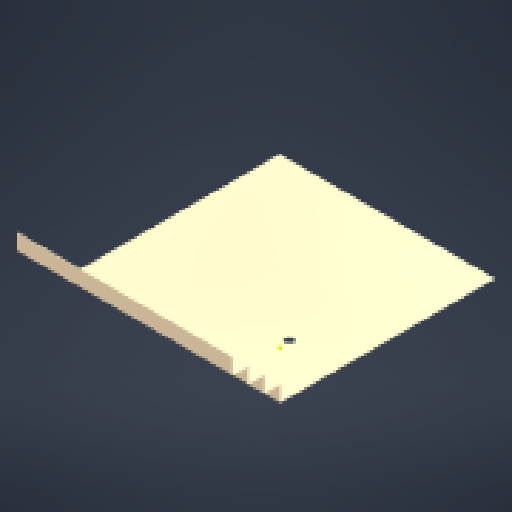
# Autodesk Inventor part: Floor, Shower
Saved by Autodesk Inventor 2026 (Build 300175000, 175)
## iProperties
Created: 2025-11-08
Part Number: Floor, Shower
Material: Polyethylene, High Density
Document SubType Name: Sheet Metal
Designer: Brandon Portillo
Density: 0.952 g/cm^3
Sheet Metal Rule: Default
Appearance: Smooth - Off-White
Author: Brandon Portillo
Autodesk Inventor part; units mm, degrees
ref_plane "YZ Plane" through (0, 0, 0) normal (1, 0, 0) x (0, 1, 0)
ref_plane "XZ Plane" through (0, 0, 0) normal (0, 1, 0) x (-1, 0, 0)
ref_plane "XY Plane" through (0, 0, 0) normal (0, 0, 1) x (1, 0, 0)
sketch "Sketch1" plane through (0, 0, 0) normal (0, 1, 0) x (-1, 0, 0)
  line L0 (0, 0) -> (1000, 0)
  line L1 (1000, 0) -> (1000, -1000)
  line L2 (1000, -1000) -> (0, -1000)
  line L3 (0, -1000) -> (0, 0)
  dimension "d0" = 1000
  dimension "d1" = 1000
  measures "d0" distance of L1.end L2.end
  measures "d1" distance of L0.end L1.end
extrude "Plate1" add sketch "Sketch1" along normal blind 3.048
sketch "Sketch2" plane through (0, 3.048, 0) normal (0, 1, 0) x (1, 0, 0)
  line L0 (-1000, 0) -> (0, 0) projected
  line L1 (0, 0) -> (-226.9109, 0)
  line L2 (-226.9109, 0) -> (-226.9109, 273.104)
  line L3 (-226.9109, 273.104) -> (0, 273.104)
  line L4 (0, 273.104) -> (0, 0)
  circle A0 centre (-226.9109, 273.104) radius 19.05
  dimension "d3" = 38.1
  constraints: 8 end point, 2 coincident, 2 parallel, 1 centre point, 1 horizontal, 1 perpendicular
  measures "d3" diameter of A0
extrude "Cut1" cut sketch "Sketch2" against normal blind 3.048 contours A0 L3 L2 | L2 L3 A0
sketch "Sketch3" plane through (0, 0, -3.048) normal (0, 0, 1) x (1, 0, 0)
  line L0 (-1000, 0) -> (0, 0)
  line L1 (0, 0) -> (0, 76.2)
  line L2 (0, 76.2) -> (-1000, 76.2)
  line L3 (-1000, 76.2) -> (-1000, 0)
  constraints: 6 end point, 1 horizontal, 1 perpendicular, 1 vertical
edge flange "Flange1" height 76.2 angle 90 thickness 3.048 bend radius 3.048 thickness toward (0, 0, 1) relief tear relief width 3.048 relief depth 1.524 edges at (-500, 3.048, 0) wall of the first edge with corners at (-1000, 0, -3.048) (0, 0, -3.048) (0, 76.2, -3.048) (-1000, 76.2, -3.048)
bend "Bend1"
corner "Corner1"
sketch "Sketch4" plane through (-1000, 73.152, -3.048) normal (0, 1, 0) x (-1, 0, 0)
  line L0 (-1000, 0) -> (0, 0)
  line L1 (0, 0) -> (0, 76.2)
  line L2 (0, 76.2) -> (-1000, 76.2)
  line L3 (-1000, 76.2) -> (-1000, 0)
  constraints: 6 end point, 1 horizontal, 1 perpendicular, 1 vertical
edge flange "Flange2" height 76.2 angle 90 thickness 3.048 bend radius 3.048 thickness toward (0, 1, 0) relief tear relief width 3.048 relief depth 1.524 edges at (-500, 76.2, 0) wall of the first edge with corners at (0, 73.152, -3.048) (-1000, 73.152, -3.048) (-1000, 73.152, 73.152) (0, 73.152, 73.152)
bend "Bend2"
corner "Corner2"
sketch "Sketch5" plane through (0, 73.152, 70.104) normal (0, 0, 1) x (1, 0, 0)
  line L0 (-1000, 0) -> (0, 0)
  line L1 (0, 0) -> (0, 76.2)
  line L2 (0, 76.2) -> (-1000, 76.2)
  line L3 (-1000, 76.2) -> (-1000, 0)
  constraints: 6 end point, 1 horizontal, 1 perpendicular, 1 vertical
edge flange "Flange3" height 76.2 angle 90 thickness 3.048 bend radius 3.048 thickness toward (0, 0, 1) relief tear relief width 3.048 relief depth 1.524 edges at (-500, 76.2, 73.152) wall of the first edge with corners at (-1000, 73.152, 70.104) (0, 73.152, 70.104) (0, 149.352, 70.104) (-1000, 149.352, 70.104)
bend "Bend3"
corner "Corner3"
sketch "Sketch6" plane through (-1000, 146.304, 70.104) normal (0, 1, 0) x (-1, 0, 0)
  line L0 (-1000, 0) -> (0, 0)
  line L1 (0, 0) -> (0, 76.2)
  line L2 (0, 76.2) -> (-1000, 76.2)
  line L3 (-1000, 76.2) -> (-1000, 0)
  constraints: 6 end point, 1 horizontal, 1 perpendicular, 1 vertical
edge flange "Flange4" height 76.2 angle 90 thickness 3.048 bend radius 3.048 thickness toward (0, 1, 0) relief tear relief width 3.048 relief depth 1.524 edges at (-500, 149.352, 73.152) wall of the first edge with corners at (0, 146.304, 70.104) (-1000, 146.304, 70.104) (-1000, 146.304, 146.304) (0, 146.304, 146.304)
bend "Bend4"
corner "Corner4"
sketch "Sketch7" plane through (0, 146.304, 143.256) normal (0, 0, 1) x (1, 0, 0)
  line L0 (-1000, 0) -> (0, 0)
  line L1 (0, 0) -> (0, 76.2)
  line L2 (0, 76.2) -> (-1000, 76.2)
  line L3 (-1000, 76.2) -> (-1000, 0)
  constraints: 6 end point, 1 horizontal, 1 perpendicular, 1 vertical
edge flange "Flange5" height 76.2 angle 90 thickness 3.048 bend radius 3.048 thickness toward (0, 0, 1) relief tear relief width 3.048 relief depth 1.524 edges at (-500, 149.352, 146.304) wall of the first edge with corners at (-1000, 146.304, 143.256) (0, 146.304, 143.256) (0, 222.504, 143.256) (-1000, 222.504, 143.256)
bend "Bend5"
corner "Corner5"
sketch "Sketch8" plane through (-1000, 222.504, 146.304) normal (0, 1, 0) x (1, 0, 0)
  point P0 (1000, 146.304)
sketch "Sketch9" plane through (-1000, 219.456, 143.256) normal (0, 1, 0) x (-1, 0, 0)
  line L0 (-1000, 0) -> (0, 0)
  line L1 (0, 0) -> (0, 76.2)
  line L2 (0, 76.2) -> (-1000, 76.2)
  line L3 (-1000, 76.2) -> (-1000, 0)
  constraints: 6 end point, 1 horizontal, 1 perpendicular, 1 vertical
edge flange "Flange6" height 76.2 angle 90 thickness 3.048 bend radius 3.048 thickness toward (0, 1, 0) relief tear relief width 3.048 relief depth 1.524 edges at (-500, 222.504, 146.304) wall of the first edge with corners at (0, 219.456, 143.256) (-1000, 219.456, 143.256) (-1000, 219.456, 219.456) (0, 219.456, 219.456)
bend "Bend6"
corner "Corner6"
sketch "Sketch10" plane through (0, 219.456, 216.408) normal (0, 0, 1) x (1, 0, 0)
  line L0 (-1000, 0) -> (0, 0)
  line L1 (0, 0) -> (0, 76.2)
  line L2 (0, 76.2) -> (-1000, 76.2)
  line L3 (-1000, 76.2) -> (-1000, 0)
  constraints: 6 end point, 1 horizontal, 1 perpendicular, 1 vertical
edge flange "Flange7" height 76.2 angle 90 thickness 3.048 bend radius 3.048 thickness toward (0, 0, 1) relief tear relief width 3.048 relief depth 1.524 edges at (-500, 222.504, 219.456) wall of the first edge with corners at (-1000, 219.456, 216.408) (0, 219.456, 216.408) (0, 295.656, 216.408) (-1000, 295.656, 216.408)
bend "Bend7"
corner "Corner7"
equation "\"d4\" = Thickness"
equation "\"d2\" = Thickness"
equation "\"d6\" = BendReliefWidth"
equation "\"d7\" = BendReliefDepth"
equation "\"d8\" = MinimumRemnant"
equation "\"d9\" = TransitionRadius"
equation "\"d12\" = BendRadius"
equation "\"d13\" = CornerReliefSize"
equation "\"d14\" = GapSize"
equation "\"d15\" = JacobiRadiusSize"
equation "\"d16\" = BendReliefWidth"
equation "\"d17\" = BendReliefDepth"
equation "\"d18\" = MinimumRemnant"
equation "\"d19\" = TransitionRadius"
equation "\"d22\" = BendRadius"
equation "\"d23\" = CornerReliefSize"
equation "\"d24\" = GapSize"
equation "\"d25\" = JacobiRadiusSize"
equation "\"d26\" = BendReliefWidth"
equation "\"d27\" = BendReliefDepth"
equation "\"d28\" = MinimumRemnant"
equation "\"d29\" = TransitionRadius"
equation "\"d32\" = BendRadius"
equation "\"d33\" = CornerReliefSize"
equation "\"d34\" = GapSize"
equation "\"d35\" = JacobiRadiusSize"
equation "\"d36\" = BendReliefWidth"
equation "\"d37\" = BendReliefDepth"
equation "\"d38\" = MinimumRemnant"
equation "\"d39\" = TransitionRadius"
equation "\"d42\" = BendRadius"
equation "\"d43\" = CornerReliefSize"
equation "\"d44\" = GapSize"
equation "\"d45\" = JacobiRadiusSize"
equation "\"d46\" = BendReliefWidth"
equation "\"d47\" = BendReliefDepth"
equation "\"d48\" = MinimumRemnant"
equation "\"d49\" = TransitionRadius"
equation "\"d52\" = BendRadius"
equation "\"d53\" = CornerReliefSize"
equation "\"d54\" = GapSize"
equation "\"d55\" = JacobiRadiusSize"
equation "\"d56\" = BendReliefWidth"
equation "\"d57\" = BendReliefDepth"
equation "\"d58\" = MinimumRemnant"
equation "\"d59\" = TransitionRadius"
equation "\"d62\" = BendRadius"
equation "\"d63\" = CornerReliefSize"
equation "\"d64\" = GapSize"
equation "\"d65\" = JacobiRadiusSize"
equation "\"d66\" = BendReliefWidth"
equation "\"d67\" = BendReliefDepth"
equation "\"d68\" = MinimumRemnant"
equation "\"d69\" = TransitionRadius"
equation "\"d72\" = BendRadius"
equation "\"d73\" = CornerReliefSize"
equation "\"d74\" = GapSize"
equation "\"d75\" = JacobiRadiusSize"
equation "\"BendRadius\" = Thickness"
equation "\"BendReliefWidth\" = Thickness"
equation "\"BendReliefDepth\" = 0.5 * Thickness"
equation "\"CornerReliefSize\" = 4 * Thickness"
equation "\"MinimumRemnant\" = 2 * Thickness"
equation "\"TransitionRadius\" = BendRadius"
equation "\"JacobiRadiusSize\" = BendRadius"
equation "\"GapSize\" = Thickness"
equation "\"Thickness\" = 3.048"
body "Solid1"
